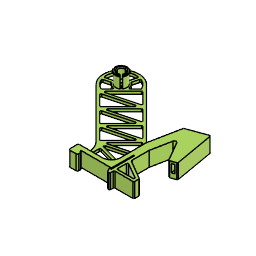
SMD_DIN (Autodesk Fusion 360 design; units mm, degrees)
Autodesk Fusion 360 part; units mm, degrees
(part 1 of 2)
sketch "スケッチ1" plane through (0, 0, 0) normal (0, 0, 1) x (1, 0, 0)
  line L0 (-17.5, 0) -> (-17.5, -1)
  line L1 (-17.5, -1) -> (-13.5, -1)
  line L2 (-13.5, -1) -> (-13.5, -7.5)
  line L3 (-13.5, -7.5) -> (13.5, -7.5)
  line L4 (-17.5, 0) -> (-12, 0)
  line L5 (-12, 0) -> (-12, -6)
  line L6 (-12, -6) -> (12, -6)
  line L7 (12, -6) -> (12, 0)
  line L8 (12, 0) -> (15.5, 0)
  line L9 (17.5, 0) -> (17.5, -1)
  line L10 (17.5, -1) -> (13.5, -1)
  line L11 (13.5, -1) -> (13.5, -7.5)
  line L12 (0, 1.75) -> (0, 22.5)
  line L13 (20, 0) -> (2.5, 0)
  line L14 (1.75, 0) -> (22.5, 0)
  line L15 (-15.5, -2.5) -> (-15.5, -4.5)
  line L16 (-17, -6) -> (-24, -6)
  line L17 (-25.5, -4.5) -> (-25.5, 16.4315)
  arc A0 (-15.5, -2.5) -> (-17, -1) centre (-17, -2.5) ccw
  arc A1 (-17, -6) -> (-15.5, -4.5) centre (-17, -4.5) ccw
  line L18 (15.5, -1.1) -> (15.5, -2.5)
  line L19 (17.5, -1.2) -> (15.7, -1.2)
  line L20 (15.5268, -1.5) -> (17.8362, -5.5)
  arc A2 (15.7, -1.2) -> (15.5268, -1.5) centre (15.7, -1.4) ccw
  line L21 (18.7022, -6) -> (19.5, -6)
  line L22 (20.5, -5) -> (20.5, -2)
  arc A3 (17.8362, -5.5) -> (18.7022, -6) centre (18.7022, -5) ccw
  arc A4 (19.5, -6) -> (20.5, -5) centre (19.5, -5) ccw
  line L23 (17.5, 0) -> (17.5, 24.5)
  line L24 (16.5, 24.5) -> (16.5, 1)
  line L25 (-12, 0) -> (12, 0)
  line L26 (21.5, -1) -> (41.5, -1)
  line L27 (20.5, 19.1658) -> (20.5, 38.2303)
  arc A5 (17.5, 24.5) -> (16.5, 24.5) centre (17, 24.5) ccw
  line L28 (15.5, 25) -> (18, 25)
  circle A6 centre (-72.5, 100) radius 6.35
  line L29 (-86.6421, 85.8579) -> (-31.3579, 30.5736)
  arc A7 (-25.5, 16.4315) -> (-31.3579, 30.5736) centre (-45.5, 16.4315) ccw
  arc A8 (-25.5, -4.5) -> (-24, -6) centre (-24, -4.5) ccw
  line L30 (-58.3579, 114.1421) -> (11.5, 44.2843)
  line L31 (48.6591, 41.9558) -> (41.1415, 39.2196)
  line L32 (41.1415, 39.2196) -> (25.8945, 65.6282)
  line L33 (25.8945, 65.6282) -> (20.5, 38.2303)
  circle A9 centre (-72.5, 100) radius 90
  line L34 (40.7244, 86.9558) -> (48.6591, 41.9558)
  line L35 (12.0723, 130.7818) -> (44.9003, 40.5877)
  line L36 (42, 5.5981) -> (21.5, 17.4338)
  line L37 (20.5, 12.815) -> (20.5, 3)
  line L38 (21.5, 2) -> (38.5, 2)
  line L39 (39, 3.866) -> (22, 13.681)
  arc A10 (38.5, 2) -> (39, 3.866) centre (38.5, 3) ccw
  arc A11 (20.5, 19.1658) -> (21.5, 17.4338) centre (22.5, 19.1658) ccw
  line L40 (17.5, -1) -> (17.5, -1.2)
  arc A12 (22, 13.681) -> (20.5, 12.815) centre (21.5, 12.815) ccw
  arc A13 (20.5, 3) -> (21.5, 2) centre (21.5, 3) ccw
  arc A14 (21.5, -1) -> (20.5, -2) centre (21.5, -2) ccw
  arc A15 (-58.3579, 114.1421) -> (-86.6421, 85.8579) centre (-72.5, 100) ccw
  line L41 (44.9003, 40.5877) -> (58.5811, 3)
  line L42 (40.7244, 86.9558) -> (18.2944, 78.792)
  line L43 (18.2944, 78.792) -> (11.5, 44.2843)
  line L44 (-25.5, 5) -> (1.5, 5)
  line L45 (11.5, 44.2843) -> (11.5, 15)
  line L46 (-54.5748, 104.7023) -> (-74.658, 84.6191)
  line L47 (-73.6921, 82.946) -> (-42.0139, 91.4342)
  line L48 (-41.5656, 93.1072) -> (-53.1606, 104.7023)
  arc A16 (-74.658, 84.6191) -> (-73.6921, 82.946) centre (-73.9509, 83.912) ccw
  arc A17 (-42.0139, 91.4342) -> (-41.5656, 93.1072) centre (-42.2727, 92.4001) ccw
  arc A18 (-53.1606, 104.7023) -> (-54.5748, 104.7023) centre (-53.8677, 103.9952) ccw
  arc A19 (1.5, 5) -> (11.5, 15) centre (1.5, 15) ccw
  circle A20 centre (-72.5, 100) radius 1.75
  arc A21 (15.5, 0) -> (16.5, 1) centre (15.5, 1) ccw
  arc A22 (4.87, 50.9143) -> (13.3114, 53.4838) centre (8.4056, 54.4498) ccw
  arc A23 (28.5593, 61.0127) -> (24.8649, 60.399) centre (26.8273, 60.0127) ccw
  line L49 (42.5, 0) -> (42.5, 4.7321)
  arc A24 (42.5, 4.7321) -> (42, 5.5981) centre (41.5, 4.7321) ccw
  arc A25 (41.5, -1) -> (42.5, 0) centre (41.5, 0) ccw
  line L50 (-52.1, 107.8842) -> (-80.3842, 79.6)
  line L51 (-80.3842, 79.6) -> (-35.77, 91.5543)
  line L52 (-35.77, 91.5543) -> (-64.0543, 63.27)
  line L53 (-74.1404, 79.7201) -> (-44.394, 87.6906)
  line L54 (-43.4281, 86.0176) -> (-62.2865, 67.1591)
  line L55 (-63.7008, 67.1591) -> (-74.5887, 78.0471)
  arc A26 (-74.1404, 79.7201) -> (-74.5887, 78.0471) centre (-73.8816, 78.7542) ccw
  arc A27 (-63.7008, 67.1591) -> (-62.2865, 67.1591) centre (-62.9936, 67.8662) ccw
  arc A28 (-43.4281, 86.0176) -> (-44.394, 87.6906) centre (-44.1352, 86.7247) ccw
  line L56 (-64.0543, 63.27) -> (-19.4401, 75.2244)
  line L57 (-19.4401, 75.2244) -> (-47.7244, 46.9401)
  line L58 (-47.7244, 46.9401) -> (-3.1102, 58.8944)
  line L59 (-3.1102, 58.8944) -> (-31.3944, 30.6102)
  line L60 (-37.5378, 87.6652) -> (-56.3963, 68.8068)
  line L61 (-55.4303, 67.1337) -> (-25.6839, 75.1043)
  line L62 (-25.2357, 76.7773) -> (-36.1236, 87.6652)
  line L63 (-57.8105, 63.3902) -> (-28.0641, 71.3607)
  line L64 (-27.0982, 69.6876) -> (-45.9566, 50.8292)
  line L65 (-47.3708, 50.8292) -> (-58.2588, 61.7171)
  line L66 (-19.7937, 71.3353) -> (-8.9057, 60.4474)
  line L67 (-9.354, 58.7743) -> (-39.1004, 50.8038)
  line L68 (-40.0663, 52.4768) -> (-21.2079, 71.3353)
  line L69 (-41.4805, 47.0602) -> (-11.7342, 55.0307)
  line L70 (-10.7682, 53.3577) -> (-29.6267, 34.4993)
  line L71 (-31.0409, 34.4993) -> (-41.9288, 45.3872)
  line L72 (-31.3944, 30.6102) -> (11.5, 42.1037)
  line L73 (-4.8779, 55.0054) -> (-23.7364, 36.1469)
  line L74 (-22.7705, 34.4739) -> (6.9759, 42.4444)
  line L75 (7.4242, 44.1174) -> (-3.4637, 55.0054)
  arc A29 (-36.1236, 87.6652) -> (-37.5378, 87.6652) centre (-36.8307, 86.9581) ccw
  arc A30 (-25.6839, 75.1043) -> (-25.2357, 76.7773) centre (-25.9428, 76.0702) ccw
  arc A31 (-56.3963, 68.8068) -> (-55.4303, 67.1337) centre (-55.6891, 68.0997) ccw
  arc A32 (-27.0982, 69.6876) -> (-28.0641, 71.3607) centre (-27.8053, 70.3947) ccw
  arc A33 (-57.8105, 63.3902) -> (-58.2588, 61.7171) centre (-57.5516, 62.4242) ccw
  arc A34 (-47.3708, 50.8292) -> (-45.9566, 50.8292) centre (-46.6637, 51.5363) ccw
  arc A35 (-19.7937, 71.3353) -> (-21.2079, 71.3353) centre (-20.5008, 70.6282) ccw
  arc A36 (-40.0663, 52.4768) -> (-39.1004, 50.8038) centre (-39.3592, 51.7697) ccw
  arc A37 (-9.354, 58.7743) -> (-8.9057, 60.4474) centre (-9.6128, 59.7403) ccw
  arc A38 (-10.7682, 53.3577) -> (-11.7342, 55.0307) centre (-11.4753, 54.0648) ccw
  arc A39 (-41.4805, 47.0602) -> (-41.9288, 45.3872) centre (-41.2217, 46.0943) ccw
  arc A40 (-31.0409, 34.4993) -> (-29.6267, 34.4993) centre (-30.3338, 35.2064) ccw
  arc A41 (-23.7364, 36.1469) -> (-22.7705, 34.4739) centre (-23.0293, 35.4398) ccw
  arc A42 (-3.4637, 55.0054) -> (-4.8779, 55.0054) centre (-4.1708, 54.2983) ccw
  arc A43 (6.9759, 42.4444) -> (7.4242, 44.1174) centre (6.7171, 43.4103) ccw
  line L76 (-22.044, 31.5627) -> (7.2412, 39.4096)
  line L77 (8.5, 38.4437) -> (8.5, 22.7499)
  line L78 (7.2412, 21.7839) -> (-22.044, 29.6309)
  arc A44 (-22.044, 31.5627) -> (-22.044, 29.6309) centre (-21.7852, 30.5968) ccw
  arc A45 (8.5, 38.4437) -> (7.2412, 39.4096) centre (7.5, 38.4437) ccw
  arc A46 (7.2412, 21.7839) -> (8.5, 22.7499) centre (7.5, 22.7499) ccw
  line L79 (-31.3579, 30.5736) -> (10.5006, 19.3577)
  line L80 (-21.5, 8) -> (1.5, 8)
  line L81 (8.5, 15) -> (8.5, 17.5735)
  line L82 (7.7588, 18.5394) -> (-21.2412, 26.3099)
  line L83 (-22.5, 25.344) -> (-22.5, 9)
  arc A47 (1.5, 8) -> (8.5, 15) centre (1.5, 15) ccw
  arc A48 (-21.2412, 26.3099) -> (-22.5, 25.344) centre (-21.5, 25.344) ccw
  arc A49 (-22.5, 9) -> (-21.5, 8) centre (-21.5, 9) ccw
  arc A50 (8.5, 17.5735) -> (7.7588, 18.5394) centre (7.5, 17.5735) ccw
  line L84 (-72.5, 100) -> (-69.2567, 96.7567)
  arc A51 (-70.7199, 116.9065) -> (-89.4065, 98.2199) centre (-72.5, 100) ccw
  arc A52 (-72.6574, 107.9985) -> (-80.4985, 100.1574) centre (-72.5, 100) ccw
  line L85 (-69.8586, 115.6532) -> (-71.7112, 108.7394)
  line L86 (-81.2394, 99.2112) -> (-88.1532, 97.3586)
  arc A53 (-69.8586, 115.6532) -> (-70.7199, 116.9065) centre (-70.8246, 115.912) ccw
  arc A54 (-72.6574, 107.9985) -> (-71.7112, 108.7394) centre (-72.6771, 108.9983) ccw
  arc A55 (-81.2394, 99.2112) -> (-80.4985, 100.1574) centre (-81.4983, 100.1771) ccw
  arc A56 (-89.4065, 98.2199) -> (-88.1532, 97.3586) centre (-88.412, 98.3246) ccw
  arc A57 (-88.0316, 93.0884) -> (-79.8094, 84.6516) centre (-72.5, 100) ccw
  arc A58 (-79.3481, 95.8644) -> (-73.6862, 92.0884) centre (-72.5, 100) ccw
  line L87 (-73.1274, 90.3924) -> (-78.6724, 84.8474)
  line L88 (-80.463, 96.3134) -> (-87.3768, 94.4609)
  line L89 (-72.5, 100) -> (-76.9533, 98.8067)
  arc A59 (-73.1274, 90.3924) -> (-73.6862, 92.0884) centre (-73.8345, 91.0995) ccw
  arc A60 (-79.3481, 95.8644) -> (-80.463, 96.3134) centre (-80.2042, 95.3475) ccw
  arc A61 (-87.3768, 94.4609) -> (-88.0316, 93.0884) centre (-87.1179, 93.4949) ccw
  arc A62 (-79.8094, 84.6516) -> (-78.6724, 84.8474) centre (-79.3795, 85.5545) ccw
  arc A63 (-57.1516, 107.3094) -> (-65.5884, 115.5316) centre (-72.5, 100) ccw
  arc A64 (-64.5884, 101.1862) -> (-68.3644, 106.8481) centre (-72.5, 100) ccw
  line L90 (-62.8924, 100.6274) -> (-57.3474, 106.1724)
  line L91 (-68.8134, 107.963) -> (-66.9609, 114.8768)
  arc A65 (-65.5884, 115.5316) -> (-66.9609, 114.8768) centre (-65.9949, 114.6179) ccw
  arc A66 (-68.8134, 107.963) -> (-68.3644, 106.8481) centre (-67.8475, 107.7042) ccw
  arc A67 (-64.5884, 101.1862) -> (-62.8924, 100.6274) centre (-63.5995, 101.3345) ccw
  arc A68 (-57.3474, 106.1724) -> (-57.1516, 107.3094) centre (-58.0545, 106.8795) ccw
  dimension "d3" = 7.5
  dimension "d4" = 1.5
  dimension "d5" = 35
  dimension "d6" = 27
  dimension "d7" = 24
  dimension "d8" = 1
  dimension "d9" = 1
  dimension "d11" = 1.5
  dimension "d12" = 1.5
  dimension "d13" = 2
  dimension "d14" = 5
  dimension "d15" = 2
  dimension "d16" = 60
  dimension "d17" = 0.2
  dimension "d18" = 0.2
  dimension "d19" = 5
  dimension "d20" = 1
  dimension "d21" = 1
  dimension "d22" = 3
  dimension "d23" = 5
  dimension "d27" = 25
  dimension "d28" = 1
  dimension "d29" = 12.7
  dimension "d30" = 55
  dimension "d31" = 100
  dimension "d33" = 135
  dimension "d34" = 20
  dimension "d35" = 10
  dimension "d36" = 1.5
  dimension "d39" = 80
  dimension "d41" = 3
  dimension "d44" = 30
  dimension "d45" = 3
  dimension "d46" = 3
  dimension "d47" = 1
  dimension "d49" = 2
  dimension "d50" = 3
  dimension "d51" = 1
  dimension "d52" = 1
  dimension "d56" = 1
  dimension "d58" = 8
  dimension "d60" = 40
  dimension "d61" = 3
  dimension "d63" = 5
  dimension "d64" = 1
  dimension "d65" = 3
  dimension "d67" = 9.35
  dimension "d68" = 30
  dimension "d77" = 10
  dimension "d100" = 3.5
  dimension "d106" = 1
  dimension "d108" = 5
  dimension "d110" = 2
  dimension "d113" = 20
  dimension "d114" = 45
  dimension "d115" = 5
  dimension "d116" = 20
  dimension "d117" = 10
  dimension "d118" = 45.6942
  dimension "d140" = 1
  dimension "d141" = 25
  dimension "d142" = 4
  dimension "d143" = 8.85
  dimension "d144" = 30
  dimension "d145" = 1.5
  dimension "d146" = 1.5
  dimension "d147" = 3
  dimension "d148" = 1
  dimension "d149" = 1.5
  dimension "d150" = 30
  dimension "d151" = 30
  dimension "d152" = 30
  dimension "d153" = 1
  dimension "d154" = 1.5
  dimension "d155" = 1.5
  dimension "d156" = 1.5
  dimension "d157" = 1.5
  dimension "d158" = 1.5
  dimension "d159" = 1.5
  dimension "d160" = 1.5
  dimension "d161" = 1.5
  dimension "d162" = 1.5
  dimension "d163" = 1.5
  dimension "d164" = 3
  dimension "d165" = 3
  dimension "d166" = 3
  dimension "d167" = 3
  dimension "d168" = 3
  dimension "d169" = 30
  dimension "d170" = 1
  dimension "d171" = 3
  dimension "d172" = 1.5
  dimension "d173" = 30
  dimension "d174" = 1.5
  dimension "d176" = 3
  dimension "d177" = 1.5
  dimension "d178" = 1
  dimension "d179" = 180
  dimension "d180" = 8
  dimension "d183" = 1
  dimension "d184" = 120
  dimension "d185" = 1.5
  dimension "d186" = 1.5
  dimension "d187" = 8
  dimension "d190" = 1
  dimension "d408" = 3
  dimension "d409" = 3
  dimension "d410" = 3
  dimension "d411" = 3
  constraint vertical L0
  constraint perpendicular L0 L1
  constraint perpendicular L1 L2
  constraint perpendicular L2 L3
  constraint perpendicular L0 L4
  constraint perpendicular L4 L5
  constraint perpendicular L5 L6
  constraint perpendicular L6 L7
  constraint perpendicular L5 L8
  constraint perpendicular L8 L9
  constraint perpendicular L5 L10
  constraint perpendicular L8 L11
  constraint symmetric L0 L9 L12
  constraint symmetric L2 L11 L12
  constraint symmetric L5 L7 L12
  constraint coincident origin L4
  constraint coincident origin L8
  constraint perpendicular L1 L15
  constraint perpendicular L15 L16
  constraint perpendicular L1 L17
  constraint tangent L15 A0
  constraint tangent L1 A0
  constraint coincident L1 A0.end
  constraint tangent L15 A1
  constraint tangent L16 A1
  constraint perpendicular L14 L18
  constraint parallel L10 L19
  constraint tangent L20 A2
  constraint tangent L19 A2
  constraint tangent L18 A2
  constraint horizontal L21
  constraint perpendicular L21 L22
  constraint tangent L20 A3
  constraint tangent L21 A3
  constraint tangent L22 A4
  constraint tangent L21 A4
  constraint perpendicular L14 L23
  constraint perpendicular L24 L25
  constraint perpendicular L22 L26
  constraint tangent L23 A5
  constraint horizontal L28
  constraint tangent A5 L28
  constraint tangent L24 A5
  constraint concentric A6 A15
  constraint tangent L29 A15
  constraint tangent L29 A7
  constraint tangent L17 A7
  constraint tangent L17 A8
  constraint tangent L16 A8
  constraint concentric A6 A9
  constraint coincident A9 L35.start
  constraint midpoint L31 L35.end
  constraint tangent A9 L35
  constraint tangent L30 A15
  constraint parallel L29 L30
  constraint vertical L37
  constraint perpendicular L37 L38
  constraint parallel L36 L39
  constraint tangent L38 A10
  constraint tangent L39 A10
  constraint tangent L27 A11
  constraint tangent L36 A11
  constraint perpendicular L19 L40
  constraint tangent L37 A12
  constraint tangent L39 A12
  constraint tangent L37 A13
  constraint tangent L38 A13
  constraint tangent L22 A14
  constraint tangent L26 A14
  constraint perpendicular L31 L41
  constraint coincident L17 L44.start
  constraint perpendicular L24 L44
  constraint perpendicular L44 L45
  constraint perpendicular L29 L46
  constraint tangent L46 A16
  constraint tangent L47 A16
  constraint tangent L48 A17
  constraint tangent L47 A17
  constraint equal A16 A17
  constraint tangent L46 A18
  constraint tangent L48 A18
  constraint equal A16 A18
  constraint tangent L45 A19
  constraint tangent L44 A19
  constraint concentric A9 A20
  constraint coincident L9.start L8
  constraint tangent L24 A21
  constraint tangent L8 A21
  constraint tangent L43 A22
  constraint tangent L30 A22
  constraint coincident L43 A22.end
  constraint coincident L30 A22.start
  constraint tangent L33 A23
  constraint tangent L32 A23
  constraint coincident L33 A23.end
  constraint coincident L32 A23.start
  constraint symmetric L34.start L35 L42.end
  constraint parallel L33 L43
  constraint perpendicular L26 L49
  constraint tangent L36 A24
  constraint tangent L49 A24
  constraint tangent L49 A25
  constraint tangent L26 A25
  constraint equal A24 A25
  constraint coincident L30 L50.start
  constraint coincident L29 L50.end
  constraint perpendicular L29 L50
  constraint coincident L30 L51.end
  constraint coincident L29 L52.end
  constraint perpendicular L29 L52
  constraint parallel L51 L53
  constraint parallel L29 L55
  constraint parallel L52 L54
  constraint tangent L53 A26
  constraint tangent L55 A26
  constraint tangent L55 A27
  constraint tangent L54 A27
  constraint equal A26 A27
  constraint tangent L54 A28
  constraint tangent L53 A28
  constraint equal A26 A28
  constraint coincident L30 L56.end
  constraint coincident L29 L57.end
  constraint perpendicular L29 L57
  constraint coincident L30 L58.end
  constraint perpendicular L30 L59
  constraint coincident L29 L59.end
  constraint coincident L45 L72.end
  constraint parallel L52 L60
  constraint parallel L56 L61
  constraint parallel L56 L63
  constraint parallel L30 L62
  constraint parallel L29 L65
  constraint parallel L57 L64
  constraint parallel L57 L68
  constraint parallel L30 L66
  constraint parallel L58 L67
  constraint parallel L29 L71
  constraint parallel L58 L69
  constraint parallel L59 L70
  constraint parallel L59 L73
  constraint parallel L30 L75
  constraint parallel L72 L74
  constraint tangent L60 A29
  constraint tangent L62 A29
  constraint tangent L62 A30
  constraint tangent L61 A30
  constraint equal A29 A30
  constraint tangent L60 A31
  constraint tangent L61 A31
  constraint equal A29 A31
  constraint tangent L63 A32
  constraint tangent L64 A32
  constraint equal A29 A32
  constraint tangent L63 A33
  constraint tangent L65 A33
  constraint equal A29 A33
  constraint tangent L64 A34
  constraint tangent L65 A34
  constraint equal A29 A34
  constraint tangent L66 A35
  constraint tangent L68 A35
  constraint equal A29 A35
  constraint tangent L67 A36
  constraint tangent L68 A36
  constraint equal A29 A36
  constraint tangent L66 A37
  constraint tangent L67 A37
  constraint equal A29 A37
  constraint tangent L69 A38
  constraint tangent L70 A38
  constraint equal A29 A38
  constraint tangent L69 A39
  constraint tangent L71 A39
  constraint equal A29 A39
  constraint tangent L70 A40
  constraint tangent L71 A40
  constraint equal A29 A40
  constraint tangent L73 A41
  constraint tangent L74 A41
  constraint equal A29 A41
  constraint tangent L73 A42
  constraint tangent L75 A42
  constraint equal A29 A42
  constraint tangent L74 A43
  constraint tangent L75 A43
  constraint equal A29 A43
  constraint parallel L72 L76
  constraint tangent L76 A44
  constraint tangent L78 A44
  constraint tangent L76 A45
  constraint tangent L77 A45
  constraint equal A44 A45
  constraint tangent L77 A46
  constraint tangent L78 A46
  constraint equal A44 A46
  constraint parallel L45 L77
  constraint coincident A19 L79.end
  constraint horizontal L80
  constraint perpendicular L80 L81
  constraint tangent L81 A47
  constraint tangent L80 A47
  constraint coincident A19.centre A47.centre
  constraint parallel L79 L82
  constraint parallel L17 L83
  constraint tangent L83 A48
  constraint tangent L82 A48
  constraint tangent L83 A49
  constraint tangent L80 A49
  constraint equal A48 A49
  constraint tangent L82 A50
  constraint tangent L81 A50
  constraint equal A48 A50
  constraint coincident A6.centre A9.centre
  constraint parallel L30 L84
  constraint symmetric L84 L85 L86
  constraint tangent A51 A53
  constraint tangent L85 A53
  constraint tangent A52 A54
  constraint tangent L85 A54
  constraint equal A53 A54
  constraint tangent A52 A55
  constraint tangent L86 A55
  constraint equal A53 A55
  constraint tangent A51 A56
  constraint tangent L86 A56
  constraint equal A53 A56
  constraint parallel L86 L89
  constraint parallel L88 L89
  constraint parallel L50 L87
  constraint tangent A58 A59
  constraint tangent L87 A59
  constraint tangent A58 A60
  constraint tangent L88 A60
  constraint equal A59 A60
  constraint tangent A57 A61
  constraint tangent L88 A61
  constraint equal A59 A61
  constraint tangent A57 A62
  constraint tangent L87 A62
  constraint equal A59 A62
  constraint symmetric L84 A57 A63
  constraint symmetric L84 A58 A64
  constraint symmetric L84 L87.start L90.start
  constraint symmetric L84 A58.end A64.start
  constraint symmetric L84 A59 A67
  constraint symmetric L84 L88.start L91.start
  constraint symmetric L84 A58.start A64.end
  constraint symmetric L84 A60 A66
  constraint symmetric L84 L88.end L91.end
  constraint symmetric L84 A57.start A63.end
  constraint symmetric L84 A61 A65
  constraint symmetric L84 L87.end L90.end
  constraint symmetric L84 A57.end A63.start
  constraint symmetric L84 A62 A68
  measures "d3" distance of L3 L14
  measures "d4" distance of L3 L6
  measures "d5" distance of L0 L9
  measures "d6" distance of L2 L11
  measures "d7" distance of L5 L7
  measures "d8" distance of L1 L4
  measures "d9" distance of L8 L10
  measures "d11" radius of A0
  measures "d12" radius of A1
  measures "d13" distance of L0 L15
  measures "d14" distance of L1 L16
  measures "d15" distance of L9 L18
  measures "d16" angle of L19 L20
  measures "d17" radius of A2
  measures "d18" distance of L10 L19
  measures "d19" distance of L10 L21
  measures "d20" radius of A3
  measures "d21" radius of A4
  measures "d22" distance of L9 L22
  measures "d23" distance of L21 L26
  measures "d27" distance of L25 L28
  measures "d28" distance of L23 L24
  measures "d29" diameter of A6
  measures "d30" distance of L0 A6.centre
  measures "d31" distance of L4 A6.centre
  measures "d33" angle of L17 L29
  measures "d34" radius of A7
  measures "d35" distance of L15 L17
  measures "d36" radius of A8
  measures "d39" angle of L25 L34
  measures "d41" distance of L23 L27
  measures "d44" angle of L26 L36
  measures "d45" distance of L26 L38
  measures "d46" distance of L36 L39
  measures "d47" radius of A10
  measures "d49" radius of A11
  measures "d50" distance of L23 L37
  measures "d51" radius of A12
  measures "d52" radius of A13
  measures "d56" radius of A14
  measures "d58" distance of L31.start L31.end
  measures "d60" distance of L35.end L41.end
  measures "d61" distance of L25 L41.end
  measures "d63" distance of L25 L44
  measures "d64" radius of A16
  measures "d65" distance of L30 L48
  measures "d67" distance of A6.centre L46
  measures "d68" angle of L46 L47
  measures "d77" radius of A19
  measures "d100" diameter of A20
  measures "d106" radius of A21
  measures "d108" radius of A22
  measures "d110" radius of A23
  measures "d113" radius of A15
  measures "d114" distance of L31 L42
  measures "d115" distance of L24 L45
  measures "d116" angle of L32 L34
  measures "d117" distance of L33 L43
  measures "d118" distance of L34.start L31.start
  measures "d140" radius of A24
  measures "d141" distance of L9 L49
  measures "d142" distance of A10.centre L49
  measures "d143" distance of A6.centre L50
  measures "d144" angle of L50 L51
  measures "d145" distance of L47 L51
  measures "d146" distance of L51 L53
  measures "d147" distance of L29 L55
  measures "d148" radius of A26
  measures "d149" distance of L52 L54
  measures "d150" angle of L52 L56
  measures "d151" angle of L57 L58
  measures "d152" angle of L59 L72
  measures "d153" radius of A29
  measures "d154" distance of L52 L60
  measures "d155" distance of L56 L61
  measures "d156" distance of L56 L63
  measures "d157" distance of L57 L64
  measures "d158" distance of L57 L68
  measures "d159" distance of L58 L67
  measures "d160" distance of L58 L69
  measures "d161" distance of L59 L70
  measures "d162" distance of L59 L73
  measures "d163" distance of L72 L74
  measures "d164" distance of L30 L62
  measures "d165" distance of L30 L66
  measures "d166" distance of L30 L75
  measures "d167" distance of L29 L71
  measures "d168" distance of L29 L65
  measures "d169" angle of L76 L78
  measures "d170" radius of A44
  measures "d171" distance of L45 L77
  measures "d172" distance of L72 L76
  measures "d173" angle of L72 L79
  measures "d174" distance of L78 L79
  measures "d176" distance of L17 L83
  measures "d177" distance of L79 L82
  measures "d178" radius of A48
  measures "d179" diameter of A9
  measures "d180" radius of A52
  measures "d183" radius of A53
  measures "d184" angle of L84 L89
  measures "d185" distance of L86 L89
  measures "d186" distance of L88 L89
  measures "d187" radius of A58
  measures "d190" radius of A59
  measures "d408" distance of L46 L87
  measures "d409" distance of A19 A47
  measures "d410" distance of A15 A57
  measures "d411" distance of A15 A51
extrude "押し出し1" add sketch "スケッチ1" along normal blind 3 contours L12 L17 A7 A9 L44 L80 L83 A49 | L12 A9 L44 L45 A19 L72 L76 L77 L78 A45 A46 L79 L80 L81 L82 A47 A50 | A7 A9 L79 L82 L83 A48 | L29 A9 L72 L76 L78 A44 L79 | L12 A9 L79 L82 | L29 L58 L59 | L30 A9 L59 L72 L73 L74 L75 A41 A42 | L30 A9 L45 L72 L74 L75 A43 | L29 L56 L57 | L30 L57 L58 | L30 L43 A22 | L29 L51 L52 | L30 L52 L56 | L29 L30 A15 L50 | L30 L50 L51 | A6 makes body 1
extrude "押し出し2" add sketch "スケッチ1" along normal blind 16.5 contours L0 L1 L4 L8 L9 L13 L14 L15 L16 L17 A0 A1 L19 L20 A2 L21 L22 A3 A4 L23 L24 L25 L26 L27 A5 A8 L31 L32 L33 L35 L36 A11 L40 A14 L42 L43 L44 L45 A19 A21 L49 A24 A25 | L31 L34 L35 L42 | L32 L33 A23 bodies 1
sketch "スケッチ2" plane through (-7.7923, 21.4092, 0) normal (0.34202, -0.939693, 0) x (0.939693, 0.34202, 0)
  line L0 (52.0743, 0) -> (60.0743, 0)
  line L1 (60.0743, 0) -> (60.0743, 16.5)
  line L2 (60.0743, 16.5) -> (52.0743, 16.5)
  line L3 (52.0743, 16.5) -> (52.0743, 0)
  line L4 (57.5743, 14.25) -> (54.5743, 14.25)
  line L5 (54.5743, 14.25) -> (54.5743, 5.25)
  line L6 (54.5743, 5.25) -> (57.5743, 5.25)
  line L7 (57.5743, 5.25) -> (57.5743, 14.25)
  line L8 (60.0743, 0) -> (52.0743, 0)
  line L9 (56.0743, 16.5) -> (56.0743, 19.1615)
  line L10 (67.6805, 9.75) -> (71.7429, 9.75)
  dimension "d78" = 9
  dimension "d80" = 3
  dimension "d111" = 6.75
  dimension "d403" = 2.5
  constraint horizontal L4
  constraint vertical L5
  constraint horizontal L6
  constraint vertical L7
  constraint midpoint L2 L9.start
  constraint perpendicular L2 L9
  constraint symmetric L5 L7 L9
  constraint perpendicular L7 L10
  constraint symmetric L4 L6 L10
  measures "d78" distance of L4 L6
  measures "d80" distance of L5 L7
  measures "d111" distance of L2 L10
  measures "d403" distance of L1 L7
sketch "スケッチ3" plane through (-23.1832, 63.6953, 0) normal (-0.34202, 0.939693, 0) x (-0.939693, -0.34202, 0)
  line L0 (-68.009, 0) -> (-44.1396, 0)
  line L1 (-44.1396, 0) -> (-44.1396, 16.5)
  line L2 (-44.1396, 16.5) -> (-68.009, 16.5)
  line L3 (-68.009, 16.5) -> (-68.009, 0)
  line L4 (-64.009, 14.9) -> (-59.009, 14.9)
  line L5 (-59.009, 14.9) -> (-59.009, 4.9)
  line L6 (-59.009, 4.9) -> (-64.009, 4.9)
  line L7 (-64.009, 4.9) -> (-64.009, 14.9)
  line L8 (-68.009, 0) -> (-44.1396, 0)
  dimension "d81" = 1.6
  dimension "d101" = 5
  dimension "d402" = 10
  dimension "d404" = 4
  constraint horizontal L4
  constraint vertical L5
  constraint horizontal L6
  constraint vertical L7
  measures "d81" distance of L2 L4
  measures "d101" distance of L5 L7
  measures "d402" distance of L4 L6
  measures "d404" distance of L3 L7
loft "ロフト1" cut profiles "スケッチ2", "スケッチ3" section 1 contours L4 L5 L6 L7 section 2 contours L4 L5 L6 L7 bodies 1
fillet "フィレット1" radius 1 4 edges at (40.7244, 86.9558, 8.25) (41.1415, 39.2196, 8.25) (48.6591, 41.9558, 8.25) (18.2944, 78.792, 8.25) on bodies 1
fillet "フィレット2" radius 1.5 1 edges at (-25.5, 5, 9.75) on bodies 1
fillet "フィレット6" radius 2 2 edges at (36.9656, 85.5877, 9.9) (32.2671, 83.8776, 9.9) on bodies 1
ref_plane "作業平面1" through (0, 100, 0) normal (0, 1, 0) x (0, 0, 1)
sketch "スケッチ4" plane through (0, 100, 0) normal (0, 1, 0) x (1, 0, 0)
  line L0 (-72.5, 1.5) -> (-72.5, -4.5)
  line L1 (-66.15, -14.7) -> (-66.15, 0)
  line L2 (-162.5, 0) -> (17.5, 0)
  line L3 (-65.35, -15.5) -> (-66.15, -14.7)
  line L4 (-65.75, -16.5) -> (-68.15, -16.5)
  line L5 (-68.15, -16.5) -> (-68.15, 0)
  line L6 (-65.75, -16.5) -> (-65.35, -16.1)
  line L7 (-65.35, -16.1) -> (-65.35, -15.5)
  dimension "d121" = 6.35
  dimension "d122" = 2
  dimension "d123" = 16.5
  dimension "d125" = 135
  dimension "d126" = 45
  dimension "d127" = 0.8
  dimension "d128" = 0.4
  dimension "d129" = 0.6
  constraint parallel L0 L1
  constraint coincident L1.end L2
  constraint perpendicular L1 L4
  constraint coincident L2 L5.end
  constraint perpendicular L2 L5
  constraint parallel L5 L7
  measures "d121" distance of L0 L1
  measures "d122" distance of L1 L5
  measures "d123" distance of L2 L4
  measures "d125" angle of L1 L3
  measures "d126" angle of L4 L6
  measures "d127" distance of L1 L7
  measures "d128" horizontal distance of L4.start L6.end
  measures "d129" distance of L3.start L6.end
revolve "回転1" add sketch "スケッチ4" angle 360 about axis through (-72.5, 100, -1.5) along (0, 0, 1) bodies 1
chamfer "面取り1" distance 1 angle 45 1 edges at (-76.5556, 98.427, 16.5) on bodies 1
sketch "スケッチ5" plane through (0, 0, 16.5) normal (0, 0, 1) x (-1, 0, 0)
  circle A0 centre (72.5, -100) radius 6.75
  circle A1 centre (72.5, -100) radius 5.35
  line L0 (72.5, -100) -> (70.3247, -97.8247)
  line L1 (58.3579, -114.1421) -> (-11.5, -44.2843)
  line L2 (70.8354, -96.9212) -> (67.9512, -94.0369)
  line L3 (69.4212, -98.3354) -> (66.5369, -95.4512)
  arc A2 (70.8354, -96.9212) -> (69.4212, -98.3354) centre (72.5, -100) ccw
  arc A3 (67.9512, -94.0369) -> (66.5369, -95.4512) centre (72.5, -100) ccw
  line L4 (72.5978, -103.4986) -> (71.5421, -107.4386)
  arc A4 (70.666, -102.981) -> (72.5978, -103.4986) centre (72.5, -100) ccw
  line L5 (70.666, -102.981) -> (69.6103, -106.9209)
  arc A5 (69.6103, -106.9209) -> (71.5421, -107.4386) centre (72.5, -100) ccw
  line L6 (75.481, -98.166) -> (79.4209, -97.1103)
  arc A6 (75.9986, -100.0978) -> (75.481, -98.166) centre (72.5, -100) ccw
  line L7 (75.9986, -100.0978) -> (79.9386, -99.0421)
  arc A7 (79.9386, -99.0421) -> (79.4209, -97.1103) centre (72.5, -100) ccw
  dimension "d132" = 2
  dimension "d133" = 3.5
  dimension "d134" = 7.5
  dimension "d136" = 360
  constraint coincident A0.centre A1.centre
  constraint parallel L0 L1
  constraint parallel L0 L3
  constraint symmetric L0 L2 L3
  constraint coincident A3 L3.end
  constraint coincident L3.end A3.end
  measures "d132" distance of L2 L3
  measures "d133" radius of A2
  measures "d134" radius of A3
extrude "押し出し3" cut sketch "スケッチ5" against normal blind 13.5 contours A0 A1 L6 L7 | A0 L6 L7 A7 | A0 L4 L5 A5 | A0 A1 L4 L5 | A1 L6 A6 L7 | A1 L4 A4 L5 | A0 A1 L2 L3 | A0 L2 L3 A3 | A1 L2 L3 A2 bodies 1
chamfer "面取り2" distance 2 angle 45 3 edges at (-68.2982, 101.1259, 3) (-73.6259, 95.7982, 3) (-75.5759, 103.0759, 3) on bodies 1
chamfer "面取り2" distance 0.6 angle 45 6 edges at (-70.1747, 104.8144, 3) (-72.1066, 105.332, 3) (-77.832, 99.6066, 3) (-77.3144, 97.6747, 3) (-68.0791, 96.9933, 3) (-69.4933, 95.5791, 3) on bodies 1
sketch "スケッチ6" plane through (0, 0, 0) normal (0, 0, 1) x (1, 0, 0)
  line L0 (-17.5, 0) -> (-17.5, -1)
  line L1 (-17.5, -1) -> (-13.5, -1)
  line L2 (-13.5, -1) -> (-13.5, -7.5)
  line L3 (-13.5, -7.5) -> (13.5, -7.5)
  line L4 (13.5, -7.5) -> (13.5, -1)
  line L5 (13.5, -1) -> (17.5, -1)
  line L6 (17.5, -1) -> (17.5, 0)
  line L7 (15.5, 0) -> (12, 0)
  line L8 (12, 0) -> (12, -6)
  line L9 (12, -6) -> (-12, -6)
  line L10 (-12, -6) -> (-12, 0)
  line L11 (-12, 0) -> (-17.5, 0)
  line L12 (0, 1.75) -> (0, 22.5)
  line L13 (20, 0) -> (2.5, 0)
  line L14 (-15, -2.5) -> (-15, -4.5)
  line L15 (-16.5, -6) -> (-19, -6)
  arc A0 (-91.8579, 104.1421) -> (-91.8579, 75.8579) centre (-77.7157, 90) ccw
  line L16 (-17.5, -1) -> (-16.5, -1)
  arc A1 (-15, -2.5) -> (-16.5, -1) centre (-16.5, -2.5) ccw
  arc A2 (-16.5, -6) -> (-15, -4.5) centre (-16.5, -4.5) ccw
  arc A3 (-21, -4) -> (-19, -6) centre (-19, -4) ccw
  line L17 (15.9, -1.2) -> (17.5, -1.2)
  line L18 (17.5, -1.2) -> (17.5, 19.5)
  line L19 (15.5536, -1.8) -> (17.6898, -5.5)
  line L20 (18.5558, -6) -> (19.5, -6)
  arc A4 (15.9, -1.2) -> (15.5536, -1.8) centre (15.9, -1.6) ccw
  arc A5 (17.6898, -5.5) -> (18.5558, -6) centre (18.5558, -5) ccw
  arc A6 (19.5, -6) -> (20.5, -5) centre (19.5, -5) ccw
  line L21 (15.5, -2.1836) -> (15.5, -1.1)
  line L22 (16.5, 1) -> (16.5, 19.5)
  arc A7 (17.5, 19.5) -> (16.5, 19.5) centre (17, 19.5) ccw
  line L23 (16.3, 20) -> (17.4, 20)
  circle A8 centre (-77.7157, 90) radius 90
  line L24 (-85.5597, 179.6575) -> (76.7844, 193.8608)
  line L25 (20.4962, 186.3107) -> (19.7989, 194.2803)
  line L26 (18.7522, 195.1918) -> (-24.2217, 193.0163)
  line L27 (-25.1674, 191.9304) -> (-23.9472, 177.9837)
  line L28 (-22.7624, 177.0888) -> (19.6886, 185.2415)
  line L29 (-91.8579, 104.1421) -> (-22.5614, 173.4386)
  line L30 (22.5, 0) -> (30, 0)
  line L31 (20.5, -5) -> (20.5, -2)
  line L32 (20.5, 10) -> (20.5, 159.4188)
  line L33 (22.5, 8) -> (26, 8)
  arc A9 (20.5, 10) -> (22.5, 8) centre (22.5, 10) ccw
  arc A10 (26, 8) -> (28, 10) centre (26, 10) ccw
  arc A11 (22.5, 0) -> (20.5, -2) centre (22.5, -2) ccw
  circle A12 centre (-77.7157, 90) radius 6.35
  circle A13 centre (-77.7157, 90) radius 1.5
  line L34 (-2.9142, 15.1985) -> (-62.2238, 74.5081)
  line L35 (-62.2238, 105.4919) -> (-2.9142, 164.8015)
  line L36 (0.5, 163.3873) -> (0.5, 16.6127)
  arc A14 (-2.9142, 15.1985) -> (0.5, 16.6127) centre (-1.5, 16.6127) ccw
  arc A15 (0.5, 163.3873) -> (-2.9142, 164.8015) centre (-1.5, 163.3873) ccw
  line L37 (19.0355, 162.9544) -> (3.1113, 178.8786)
  arc A16 (-22.5614, 173.4386) -> (-22.5614, 176.267) centre (-23.9756, 174.8528) ccw
  arc A17 (4.1483, 182.257) -> (3.1113, 178.8786) centre (4.5255, 180.2929) ccw
  line L38 (-21, -4) -> (-21, 5)
  line L39 (-91.8579, 75.8579) -> (-21, 5)
  arc A18 (20.5, 159.4188) -> (19.0355, 162.9544) centre (15.5, 159.4188) ccw
  line L40 (-21, 5) -> (8.5, 5)
  line L41 (13.5, 10) -> (13.5, 19.5)
  arc A19 (8.5, 5) -> (13.5, 10) centre (8.5, 10) ccw
  line L42 (12, 0) -> (-12, 0)
  arc A20 (51.3253, 16.25) -> (28, 10) centre (40.5, 10) ccw
  arc A21 (20.5, 19.5) -> (13.5, 19.5) centre (17, 19.5) ccw
  arc A22 (-62.3465, 77.2021) -> (-62.3465, 102.7979) centre (-77.7157, 90) ccw
  arc A23 (-62.3465, 77.2021) -> (-62.2238, 74.5081) centre (-60.8096, 75.9223) ccw
  arc A24 (-62.2238, 105.4919) -> (-62.3465, 102.7979) centre (-60.8096, 104.0777) ccw
  arc A25 (-88.2594, 100.7647) -> (-88.2594, 79.2353) centre (-77.7157, 90) ccw
  arc A26 (-84.2941, 95.1427) -> (-84.2941, 84.8573) centre (-77.7157, 90) ccw
  line L43 (-86.6937, 79.4497) -> (-84.2159, 83.7414)
  line L44 (-86.6937, 100.5503) -> (-84.2159, 96.2586)
  line L45 (-77.7157, 90) -> (-79.5324, 86.8534)
  line L46 (-77.7157, 90) -> (-81.3326, 90)
  arc A27 (-86.6937, 100.5503) -> (-88.2594, 100.7647) centre (-87.5597, 100.0503) ccw
  arc A28 (-84.2941, 95.1427) -> (-84.2159, 96.2586) centre (-85.0819, 95.7586) ccw
  arc A29 (-88.2594, 79.2353) -> (-86.6937, 79.4497) centre (-87.5597, 79.9497) ccw
  arc A30 (-84.2159, 83.7414) -> (-84.2941, 84.8573) centre (-85.0819, 84.2414) ccw
  arc A31 (-78.8803, 81.7316) -> (-69.9728, 86.8743) centre (-77.7157, 90) ccw
  line L47 (-82.3636, 76.9497) -> (-79.8858, 81.2414)
  arc A32 (-81.7663, 75.4865) -> (-63.1214, 86.2512) centre (-77.7157, 90) ccw
  line L48 (-64.09, 87.5) -> (-69.0455, 87.5)
  arc A33 (-63.1214, 86.2512) -> (-64.09, 87.5) centre (-64.09, 86.5) ccw
  arc A34 (-69.0455, 87.5) -> (-69.9728, 86.8743) centre (-69.0455, 86.5) ccw
  arc A35 (-78.8803, 81.7316) -> (-79.8858, 81.2414) centre (-79.0197, 80.7414) ccw
  arc A36 (-82.3636, 76.9497) -> (-81.7663, 75.4865) centre (-81.4975, 76.4497) ccw
  arc A37 (-69.9728, 93.1257) -> (-78.8803, 98.2684) centre (-77.7157, 90) ccw
  line L49 (-64.09, 92.5) -> (-69.0455, 92.5)
  arc A38 (-63.1214, 93.7488) -> (-81.7663, 104.5135) centre (-77.7157, 90) ccw
  line L50 (-82.3636, 103.0503) -> (-79.8858, 98.7586)
  arc A39 (-81.7663, 104.5135) -> (-82.3636, 103.0503) centre (-81.4975, 103.5503) ccw
  arc A40 (-79.8858, 98.7586) -> (-78.8803, 98.2684) centre (-79.0197, 99.2586) ccw
  arc A41 (-69.9728, 93.1257) -> (-69.0455, 92.5) centre (-69.0455, 93.5) ccw
  arc A42 (-64.09, 92.5) -> (-63.1214, 93.7488) centre (-64.09, 93.5) ccw
  line L51 (33, 3) -> (33, 10)
  arc A43 (46.9952, 13.75) -> (51.3253, 16.25) centre (49.1603, 15) ccw
  arc A44 (46.9952, 13.75) -> (33, 10) centre (40.5, 10) ccw
  arc A45 (30, 0) -> (33, 3) centre (30, 3) ccw
  line L52 (40.5, 10) -> (45.9092, 13.123)
  arc A46 (15.5, 0) -> (16.5, 1) centre (15.5, 1) ccw
  line L53 (40.5, 10) -> (40.4841, 10)
  line L54 (0.5, 90) -> (-52.75, 36.75)
  line L55 (-52.75, 36.75) -> (-52.75, 65.0343)
  line L56 (-52.75, 65.0343) -> (-66.8921, 50.8921)
  line L57 (-66.8921, 50.8921) -> (-66.8921, 79.1764)
  line L58 (-66.8921, 79.1764) -> (-81.0343, 65.0343)
  line L59 (-55.9571, 44.1997) -> (-63.003, 51.2457)
  line L60 (-63.003, 52.6599) -> (-55.9571, 59.7058)
  line L61 (-54.25, 58.9987) -> (-54.25, 44.9069)
  arc A47 (-63.003, 52.6599) -> (-63.003, 51.2457) centre (-62.2959, 51.9528) ccw
  arc A48 (-54.25, 58.9987) -> (-55.9571, 59.7058) centre (-55.25, 58.9987) ccw
  arc A49 (-55.9571, 44.1997) -> (-54.25, 44.9069) centre (-55.25, 44.9069) ccw
  line L62 (-51.25, 42.7855) -> (-51.25, 56.8774)
  line L63 (-49.5429, 57.5845) -> (-42.497, 50.5386)
  line L64 (-42.497, 49.1244) -> (-49.5429, 42.0784)
  arc A50 (-51.25, 42.7855) -> (-49.5429, 42.0784) centre (-50.25, 42.7855) ccw
  arc A51 (-49.5429, 57.5845) -> (-51.25, 56.8774) centre (-50.25, 56.8774) ccw
  arc A52 (-42.497, 49.1244) -> (-42.497, 50.5386) centre (-43.2041, 49.8315) ccw
  line L65 (-38.6079, 50.8921) -> (-38.6079, 22.6079)
  line L66 (-38.6079, 22.6079) -> (-24.4657, 36.75)
  line L67 (-63.685, 56.2206) -> (-56.6391, 63.2665)
  line L68 (-56.6391, 64.6807) -> (-63.685, 71.7267)
  line L69 (-65.3921, 71.0196) -> (-65.3921, 56.9277)
  arc A53 (-65.3921, 56.9277) -> (-63.685, 56.2206) centre (-64.3921, 56.9277) ccw
  arc A54 (-63.685, 71.7267) -> (-65.3921, 71.0196) centre (-64.3921, 71.0196) ccw
  arc A55 (-56.6391, 63.2665) -> (-56.6391, 64.6807) centre (-57.3462, 63.9736) ccw
  line L70 (-70.0992, 58.3419) -> (-77.1452, 65.3878)
  line L71 (-77.1452, 66.802) -> (-70.0992, 73.848)
  line L72 (-68.3921, 73.1409) -> (-68.3921, 59.049)
  arc A56 (-70.0992, 58.3419) -> (-68.3921, 59.049) centre (-69.3921, 59.049) ccw
  arc A57 (-77.1452, 66.802) -> (-77.1452, 65.3878) centre (-76.4381, 66.0949) ccw
  arc A58 (-68.3921, 73.1409) -> (-70.0992, 73.848) centre (-69.3921, 73.1409) ccw
  line L73 (-24.4657, 36.75) -> (-24.4657, 8.4657)
  line L74 (-24.4657, 8.4657) -> (-10.3236, 22.6079)
  line L75 (-10.3236, 22.6079) -> (-10.3236, 5)
  line L76 (-22.9657, 14.5013) -> (-22.9657, 28.5931)
  line L77 (-21.2586, 29.3003) -> (-14.2127, 22.2543)
  line L78 (-14.2127, 20.8401) -> (-21.2586, 13.7942)
  line L79 (-27.6728, 15.9155) -> (-34.7188, 22.9614)
  line L80 (-34.7188, 24.3756) -> (-27.6728, 31.4216)
  line L81 (-25.9657, 30.7145) -> (-25.9657, 16.6226)
  line L82 (-37.1079, 28.6434) -> (-37.1079, 42.7353)
  line L83 (-35.4008, 43.4424) -> (-28.3548, 36.3964)
  line L84 (-28.3548, 34.9822) -> (-35.4008, 27.9363)
  line L85 (-48.8609, 37.1036) -> (-41.815, 30.0576)
  line L86 (-40.1079, 30.7647) -> (-40.1079, 44.8566)
  line L87 (-41.815, 45.5637) -> (-48.8609, 38.5178)
  arc A59 (-48.8609, 38.5178) -> (-48.8609, 37.1036) centre (-48.1538, 37.8107) ccw
  arc A60 (-40.1079, 44.8566) -> (-41.815, 45.5637) centre (-41.1079, 44.8566) ccw
  arc A61 (-41.815, 30.0576) -> (-40.1079, 30.7647) centre (-41.1079, 30.7647) ccw
  arc A62 (-37.1079, 28.6434) -> (-35.4008, 27.9363) centre (-36.1079, 28.6434) ccw
  arc A63 (-35.4008, 43.4424) -> (-37.1079, 42.7353) centre (-36.1079, 42.7353) ccw
  arc A64 (-28.3548, 34.9822) -> (-28.3548, 36.3964) centre (-29.0619, 35.6893) ccw
  arc A65 (-34.7188, 24.3756) -> (-34.7188, 22.9614) centre (-34.0117, 23.6685) ccw
  arc A66 (-27.6728, 15.9155) -> (-25.9657, 16.6226) centre (-26.9657, 16.6226) ccw
  arc A67 (-25.9657, 30.7145) -> (-27.6728, 31.4216) centre (-26.9657, 30.7145) ccw
  arc A68 (-21.2586, 29.3003) -> (-22.9657, 28.5931) centre (-21.9657, 28.5931) ccw
  arc A69 (-22.9657, 14.5013) -> (-21.2586, 13.7942) centre (-21.9657, 14.5013) ccw
  arc A70 (-14.2127, 20.8401) -> (-14.2127, 22.2543) centre (-14.9198, 21.5472) ccw
  line L88 (-21.103, 9.7071) -> (-13.5307, 17.2794)
  line L89 (-11.8236, 16.5723) -> (-11.8236, 9)
  line L90 (-12.8236, 8) -> (-20.3959, 8)
  arc A71 (-21.103, 9.7071) -> (-20.3959, 8) centre (-20.3959, 9) ccw
  arc A72 (-12.8236, 8) -> (-11.8236, 9) centre (-12.8236, 9) ccw
  arc A73 (-11.8236, 16.5723) -> (-13.5307, 17.2794) centre (-12.8236, 16.5723) ccw
  line L91 (-8.8236, 9) -> (-8.8236, 14.451)
  line L92 (-7.1165, 15.1581) -> (-1.6655, 9.7071)
  line L93 (-2.3726, 8) -> (-7.8236, 8)
  arc A74 (-8.8236, 9) -> (-7.8236, 8) centre (-7.8236, 9) ccw
  arc A75 (-7.1165, 15.1581) -> (-8.8236, 14.451) centre (-7.8236, 14.451) ccw
  arc A76 (-2.3726, 8) -> (-1.6655, 9.7071) centre (-2.3726, 9) ccw
  line L94 (-70.0992, 121.6581) -> (-77.1452, 114.6122)
  line L95 (-77.1452, 113.198) -> (-70.0992, 106.152)
  arc A77 (-70.0992, 106.152) -> (-68.3921, 106.8591) centre (-69.3921, 106.8591) ccw
  line L96 (-68.3921, 106.8591) -> (-68.3921, 120.951)
  arc A78 (-68.3921, 120.951) -> (-70.0992, 121.6581) centre (-69.3921, 120.951) ccw
  arc A79 (-77.1452, 114.6122) -> (-77.1452, 113.198) centre (-76.4381, 113.9051) ccw
  arc A80 (-65.3921, 108.9804) -> (-63.685, 108.2733) centre (-64.3921, 108.9804) ccw
  line L97 (-65.3921, 108.9804) -> (-65.3921, 123.0723)
  arc A81 (-63.685, 123.7794) -> (-65.3921, 123.0723) centre (-64.3921, 123.0723) ccw
  line L98 (-63.685, 123.7794) -> (-56.6391, 116.7335)
  line L99 (-56.6391, 115.3193) -> (-63.685, 108.2733)
  arc A82 (-56.6391, 115.3193) -> (-56.6391, 116.7335) centre (-57.3462, 116.0264) ccw
  arc A83 (-54.25, 135.0931) -> (-55.9571, 135.8003) centre (-55.25, 135.0931) ccw
  line L100 (-55.9571, 135.8003) -> (-63.003, 128.7543)
  line L101 (-54.25, 121.0013) -> (-54.25, 135.0931)
  arc A84 (-55.9571, 120.2942) -> (-54.25, 121.0013) centre (-55.25, 121.0013) ccw
  line L102 (-63.003, 127.3401) -> (-55.9571, 120.2942)
  arc A85 (-63.003, 128.7543) -> (-63.003, 127.3401) centre (-62.2959, 128.0472) ccw
  arc A86 (-49.5429, 137.9216) -> (-51.25, 137.2145) centre (-50.25, 137.2145) ccw
  line L103 (-51.25, 137.2145) -> (-51.25, 123.1226)
  line L104 (-42.497, 130.8756) -> (-49.5429, 137.9216)
  line L105 (-49.5429, 122.4155) -> (-42.497, 129.4614)
  arc A87 (-42.497, 129.4614) -> (-42.497, 130.8756) centre (-43.2041, 130.1685) ccw
  arc A88 (-51.25, 123.1226) -> (-49.5429, 122.4155) centre (-50.25, 123.1226) ccw
  arc A89 (-48.8609, 142.8964) -> (-48.8609, 141.4822) centre (-48.1538, 142.1893) ccw
  line L106 (-48.8609, 142.8964) -> (-41.815, 149.9424)
  line L107 (-41.815, 134.4363) -> (-48.8609, 141.4822)
  line L108 (-40.1079, 149.2353) -> (-40.1079, 135.1434)
  arc A90 (-41.815, 134.4363) -> (-40.1079, 135.1434) centre (-41.1079, 135.1434) ccw
  arc A91 (-40.1079, 149.2353) -> (-41.815, 149.9424) centre (-41.1079, 149.2353) ccw
  arc A92 (-35.4008, 152.0637) -> (-37.1079, 151.3566) centre (-36.1079, 151.3566) ccw
  line L109 (-37.1079, 151.3566) -> (-37.1079, 137.2647)
  line L110 (-28.3548, 145.0178) -> (-35.4008, 152.0637)
  arc A93 (-28.3548, 143.6036) -> (-28.3548, 145.0178) centre (-29.0619, 144.3107) ccw
  line L111 (-35.4008, 136.5576) -> (-28.3548, 143.6036)
  arc A94 (-37.1079, 137.2647) -> (-35.4008, 136.5576) centre (-36.1079, 137.2647) ccw
  line L112 (-27.6728, 164.0845) -> (-34.7188, 157.0386)
  arc A95 (-25.9657, 163.3774) -> (-27.6728, 164.0845) centre (-26.9657, 163.3774) ccw
  line L113 (-25.9657, 149.2855) -> (-25.9657, 163.3774)
  arc A96 (-27.6728, 148.5784) -> (-25.9657, 149.2855) centre (-26.9657, 149.2855) ccw
  line L114 (-34.7188, 155.6244) -> (-27.6728, 148.5784)
  arc A97 (-34.7188, 157.0386) -> (-34.7188, 155.6244) centre (-34.0117, 156.3315) ccw
  line L115 (-22.9657, 165.4987) -> (-22.9657, 151.4069)
  line L116 (-14.2127, 159.1599) -> (-21.2586, 166.2058)
  arc A98 (-21.2586, 166.2058) -> (-22.9657, 165.4987) centre (-21.9657, 165.4987) ccw
  line L117 (-21.2586, 150.6997) -> (-14.2127, 157.7457)
  arc A99 (-22.9657, 151.4069) -> (-21.2586, 150.6997) centre (-21.9657, 151.4069) ccw
  arc A100 (-14.2127, 157.7457) -> (-14.2127, 159.1599) centre (-14.9198, 158.4528) ccw
  line L118 (-24.4657, 171.5343) -> (-10.3236, 157.3921)
  line L119 (-19.1373, 168.3272) -> (-12.0914, 161.2812)
  line L120 (-10.6771, 161.2812) -> (-3.6312, 168.3272)
  line L121 (-4.3383, 170.0343) -> (-18.4302, 170.0343)
  arc A101 (-12.0914, 161.2812) -> (-10.6771, 161.2812) centre (-11.3843, 161.9883) ccw
  arc A102 (-18.4302, 170.0343) -> (-19.1373, 168.3272) centre (-18.4302, 169.0343) ccw
  arc A103 (-3.6312, 168.3272) -> (-4.3383, 170.0343) centre (-4.3383, 169.0343) ccw
  line L122 (-1.5, 174.0343) -> (-1.5, 176.9071)
  line L123 (-2.6886, 177.8891) -> (-17.6472, 175.0163)
  line L124 (-17.4586, 173.0343) -> (-2.5, 173.0343)
  arc A104 (-17.6472, 175.0163) -> (-17.4586, 173.0343) centre (-17.4586, 174.0343) ccw
  arc A105 (-2.5, 173.0343) -> (-1.5, 174.0343) centre (-2.5, 174.0343) ccw
  arc A106 (-1.5, 176.9071) -> (-2.6886, 177.8891) centre (-2.5, 176.9071) ccw
  line L125 (0.5, 90) -> (20.5, 90)
  line L126 (20.5, 90) -> (0.5, 110)
  line L127 (0.5, 110) -> (20.5, 110)
  line L128 (20.5, 110) -> (0.5, 130)
  line L129 (0.5, 130) -> (20.5, 130)
  line L130 (20.5, 130) -> (0.5, 150)
  line L131 (0.5, 150) -> (20.5, 150)
  line L132 (20.5, 150) -> (0.8621, 169.6379)
  line L133 (3.5, 92.5) -> (3.5, 102.4645)
  line L134 (5.2071, 103.1716) -> (15.1716, 93.2071)
  line L135 (14.4645, 91.5) -> (4.5, 91.5)
  line L136 (5.8284, 106.7929) -> (15.7929, 96.8284)
  line L137 (17.5, 97.5355) -> (17.5, 107.5)
  line L138 (16.5, 108.5) -> (6.5355, 108.5)
  arc A107 (5.2071, 103.1716) -> (3.5, 102.4645) centre (4.5, 102.4645) ccw
  arc A108 (3.5, 92.5) -> (4.5, 91.5) centre (4.5, 92.5) ccw
  arc A109 (14.4645, 91.5) -> (15.1716, 93.2071) centre (14.4645, 92.5) ccw
  arc A110 (15.7929, 96.8284) -> (17.5, 97.5355) centre (16.5, 97.5355) ccw
  arc A111 (6.5355, 108.5) -> (5.8284, 106.7929) centre (6.5355, 107.5) ccw
  arc A112 (17.5, 107.5) -> (16.5, 108.5) centre (16.5, 107.5) ccw
  arc A113 (3.5, 112.5) -> (4.5, 111.5) centre (4.5, 112.5) ccw
  arc A114 (14.4645, 111.5) -> (15.1716, 113.2071) centre (14.4645, 112.5) ccw
  line L139 (14.4645, 111.5) -> (4.5, 111.5)
  line L140 (5.2071, 123.1716) -> (15.1716, 113.2071)
  arc A115 (5.2071, 123.1716) -> (3.5, 122.4645) centre (4.5, 122.4645) ccw
  line L141 (3.5, 112.5) -> (3.5, 122.4645)
  line L142 (5.8284, 126.7929) -> (15.7929, 116.8284)
  arc A116 (6.5355, 128.5) -> (5.8284, 126.7929) centre (6.5355, 127.5) ccw
  line L143 (16.5, 128.5) -> (6.5355, 128.5)
  line L144 (17.5, 117.5355) -> (17.5, 127.5)
  arc A117 (17.5, 127.5) -> (16.5, 128.5) centre (16.5, 127.5) ccw
  arc A118 (15.7929, 116.8284) -> (17.5, 117.5355) centre (16.5, 117.5355) ccw
  arc A119 (3.5, 132.5) -> (4.5, 131.5) centre (4.5, 132.5) ccw
  arc A120 (14.4645, 131.5) -> (15.1716, 133.2071) centre (14.4645, 132.5) ccw
  line L145 (14.4645, 131.5) -> (4.5, 131.5)
  line L146 (5.2071, 143.1716) -> (15.1716, 133.2071)
  arc A121 (5.2071, 143.1716) -> (3.5, 142.4645) centre (4.5, 142.4645) ccw
  line L147 (3.5, 132.5) -> (3.5, 142.4645)
  line L148 (5.8284, 146.7929) -> (15.7929, 136.8284)
  arc A122 (6.5355, 148.5) -> (5.8284, 146.7929) centre (6.5355, 147.5) ccw
  line L149 (16.5, 148.5) -> (6.5355, 148.5)
  line L150 (17.5, 137.5355) -> (17.5, 147.5)
  arc A123 (17.5, 147.5) -> (16.5, 148.5) centre (16.5, 147.5) ccw
  arc A124 (15.7929, 136.8284) -> (17.5, 137.5355) centre (16.5, 137.5355) ccw
  line L151 (4.5, 151.5) -> (14.4645, 151.5)
  line L152 (15.1716, 153.2071) -> (5.2071, 163.1716)
  line L153 (3.5, 162.4645) -> (3.5, 152.5)
  arc A125 (3.5, 152.5) -> (4.5, 151.5) centre (4.5, 152.5) ccw
  arc A126 (5.2071, 163.1716) -> (3.5, 162.4645) centre (4.5, 162.4645) ccw
  arc A127 (14.4645, 151.5) -> (15.1716, 153.2071) centre (14.4645, 152.5) ccw
  line L154 (3.5, 87.5) -> (3.5, 77.5355)
  arc A128 (4.5, 88.5) -> (3.5, 87.5) centre (4.5, 87.5) ccw
  line L155 (14.4645, 88.5) -> (4.5, 88.5)
  line L156 (5.2071, 76.8284) -> (15.1716, 86.7929)
  arc A129 (3.5, 77.5355) -> (5.2071, 76.8284) centre (4.5, 77.5355) ccw
  arc A130 (15.1716, 86.7929) -> (14.4645, 88.5) centre (14.4645, 87.5) ccw
  line L157 (5.8284, 73.2071) -> (15.7929, 83.1716)
  arc A131 (17.5, 82.4645) -> (15.7929, 83.1716) centre (16.5, 82.4645) ccw
  line L158 (17.5, 82.4645) -> (17.5, 72.5)
  arc A132 (16.5, 71.5) -> (17.5, 72.5) centre (16.5, 72.5) ccw
  line L159 (16.5, 71.5) -> (6.5355, 71.5)
  arc A133 (5.8284, 73.2071) -> (6.5355, 71.5) centre (6.5355, 72.5) ccw
  line L160 (3.5, 67.5) -> (3.5, 57.5355)
  arc A134 (4.5, 68.5) -> (3.5, 67.5) centre (4.5, 67.5) ccw
  arc A135 (3.5, 57.5355) -> (5.2071, 56.8284) centre (4.5, 57.5355) ccw
  line L161 (5.2071, 56.8284) -> (15.1716, 66.7929)
  arc A136 (15.1716, 66.7929) -> (14.4645, 68.5) centre (14.4645, 67.5) ccw
  line L162 (14.4645, 68.5) -> (4.5, 68.5)
  line L163 (16.5, 51.5) -> (6.5355, 51.5)
  arc A137 (5.8284, 53.2071) -> (6.5355, 51.5) centre (6.5355, 52.5) ccw
  line L164 (5.8284, 53.2071) -> (15.7929, 63.1716)
  arc A138 (17.5, 62.4645) -> (15.7929, 63.1716) centre (16.5, 62.4645) ccw
  line L165 (17.5, 62.4645) -> (17.5, 52.5)
  arc A139 (16.5, 51.5) -> (17.5, 52.5) centre (16.5, 52.5) ccw
  arc A140 (15.1716, 46.7929) -> (14.4645, 48.5) centre (14.4645, 47.5) ccw
  line L166 (14.4645, 48.5) -> (4.5, 48.5)
  arc A141 (3.5, 37.5355) -> (5.2071, 36.8284) centre (4.5, 37.5355) ccw
  line L167 (3.5, 47.5) -> (3.5, 37.5355)
  arc A142 (4.5, 48.5) -> (3.5, 47.5) centre (4.5, 47.5) ccw
  line L168 (5.2071, 36.8284) -> (15.1716, 46.7929)
  arc A143 (5.8284, 33.2071) -> (6.5355, 31.5) centre (6.5355, 32.5) ccw
  line L169 (16.5, 31.5) -> (6.5355, 31.5)
  line L170 (5.8284, 33.2071) -> (15.7929, 43.1716)
  arc A144 (17.5, 42.4645) -> (15.7929, 43.1716) centre (16.5, 42.4645) ccw
  line L171 (17.5, 42.4645) -> (17.5, 32.5)
  arc A145 (16.5, 31.5) -> (17.5, 32.5) centre (16.5, 32.5) ccw
  line L172 (15.1716, 26.7929) -> (5.2071, 16.8284)
  arc A146 (15.1716, 26.7929) -> (14.4645, 28.5) centre (14.4645, 27.5) ccw
  line L173 (4.5, 28.5) -> (14.4645, 28.5)
  line L174 (3.5, 17.5355) -> (3.5, 27.5)
  arc A147 (3.5, 17.5355) -> (5.2071, 16.8284) centre (4.5, 17.5355) ccw